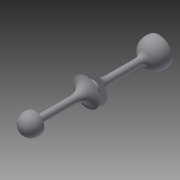
# Autodesk Inventor part: Fish Vertebrae
Saved by Autodesk Inventor 2015 (Build 190159000, 159)
## iProperties
Created: 2014-11-02
Part Number: Fish Vertebrae
Material: Generic
Document SubType Name: Modeling
Designer: Ryan
Density: 1 g/cm^3
Appearance: Default
Mass: 0.782179 g
Surface Area: 11.0524 cm^2
Volume: 0.782179 cm^3
Author: Ryan
Autodesk Inventor part; units mm, degrees
ref_plane "YZ Plane" through (0, 0, 0) normal (1, 0, 0) x (0, 1, 0)
ref_plane "XZ Plane" through (0, 0, 0) normal (0, 1, 0) x (-1, 0, 0)
ref_plane "XY Plane" through (0, 0, 0) normal (0, 0, 1) x (1, 0, 0)
sketch "Sketch1" plane through (0, 0, 0) normal (1, 0, 0) x (0, 1, 0)
  arc A0 (3.5921, 20.32) -> (0, 25.4) centre (0, 21.59) ccw
  arc A1 (3.5921, -25.4) -> (0, -20.32) centre (0, -24.13) ccw
  line L0 (4.9187, -25.4) -> (3.5921, -25.4)
  line L1 (0, 21.59) -> (0, 25.4)
  line L2 (1.27, 17.9531) -> (1.27, 6.4568)
  arc A2 (3.5921, 20.32) -> (1.27, 17.9531) centre (3.6374, 17.9531) ccw
  line L3 (2.54, 1.27) -> (2.54, -1.27)
  line L4 (5.08, -1.27) -> (2.54, -1.27)
  line L5 (5.08, 1.27) -> (2.54, 1.27)
  arc A3 (4.9187, -25.4) -> (2.4811, -19.6971) centre (0, -24.13) ccw
  line L6 (0, 0) -> (0, -20.32)
  line L7 (0, 0) -> (0, 21.59)
  line L8 (1.27, -6.4568) -> (1.27, -17.6313)
  arc A4 (1.27, -17.6313) -> (2.4811, -19.6971) centre (3.6374, -17.6313) ccw
  arc A5 (1.27, 6.4568) -> (5.08, 1.27) centre (6.7056, 6.4568) ccw
  arc A6 (5.08, -1.27) -> (1.27, -6.4568) centre (6.7056, -6.4568) ccw
  dimension "d7" = 7.62
  dimension "d9" = 7.62
  dimension "d17" = 1.27
  dimension "d18" = 1.27
  dimension "d19" = 2.54
  dimension "d21" = 25.4
  dimension "d22" = 25.4
  dimension "d23" = 1.27
  dimension "d24" = 1.27
  dimension "d25" = 5.08
  dimension "d26" = 5.08
  dimension "d27" = 5.08
  constraints: 18 end point, 14 point on circle, 7 centre point, 5 tangent, 4 vertical, 3 vertical alignment, 2 horizontal, 1 coincident, 1 collinear, 1 parallel, 1 point on line
  measures "d7" diameter of A0
  measures "d9" diameter of A1
  measures "d17" vertical distance of L6.start L3.start
  measures "d18" vertical distance of L3.end L6.start
  measures "d19" distance between parallel lines of L7 L3
  measures "d21" distance of L1.end L6.start
  measures "d22" distance from line of L6.start L0
  measures "d23" distance between parallel lines of L7 L2
  measures "d24" radial gap between concentric circles of A1 A3
  measures "d25" vertical distance of L6.end L0.end
  measures "d26" vertical distance of L1.end A0.start
  measures "d27" distance from line of L6 L4.start
revolve "Revolution1" add sketch "Sketch1" angle 360 about axis through (0, 0, 0) along (0, 0, 1)
body "Solid1"
